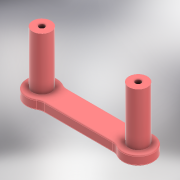
# Autodesk Inventor part: BRAÇO ROBÓTICO - Garra A2b - Pino
Saved by Autodesk Inventor 2021 (Build 250183000, 183)
## iProperties
Created: 2020-08-23
Part Number: BRAÇO ROBÓTICO - Garra A2b - Pino
Material: Plástico PC/ABS
Document SubType Name: Modeling
Designer: Araújo, I.
Mass: 0.348924 g
Surface Area: 10.9374 cm^2
Volume: 0.976633 cm^3
Density: 0.357273 g/cm^3
Appearance: Liso - Branco
Author: Araújo, I.
## iProperties of the stored document _3DPrint.ipt
Created: 2020-11-23
Part Number: _3DPrint
Material: Genérico
Document SubType Name: Modeling
Designer: Araújo, I.
Mass: 0.976633 g
Surface Area: 10.9374 cm^2
Volume: 0.976633 cm^3
Density: 1 g/cm^3
Appearance: Padrão
Author: Araújo, I.
Autodesk Inventor part; units mm, degrees
ref_plane "YZ Plane" through (0, 0, 0) normal (1, 0, 0) x (0, 1, 0)
ref_plane "XZ Plane" through (0, 0, 0) normal (0, 1, 0) x (-1, 0, 0)
ref_plane "XY Plane" through (0, 0, 0) normal (0, 0, 1) x (1, 0, 0)
sketch "Esboço1" plane through (0, 0, 0) normal (0, 1, 0) x (-1, 0, 0)
  arc A0 (-2.0603, -3.4286) -> (-2.0603, 3.4286) centre (0, 0) ccw
  arc A1 (-22.9397, 3.4286) -> (-22.9397, -3.4286) centre (-25, 0) ccw
  line L0 (-3.6056, -3) -> (-21.3944, -3)
  line L1 (-3.6056, 3) -> (-21.3944, 3)
  arc A2 (-2.0603, -3.4286) -> (-3.6056, -3) centre (-3.6056, -6) ccw
  arc A3 (-3.6056, 3) -> (-2.0603, 3.4286) centre (-3.6056, 6) ccw
  arc A4 (-21.3944, -3) -> (-22.9397, -3.4286) centre (-21.3944, -6) ccw
  arc A5 (-22.9397, 3.4286) -> (-21.3944, 3) centre (-21.3944, 6) ccw
  point P0 (-2.6458, -3)
  point P1 (-22.3542, -3)
  point P2 (-2.6458, 3)
  point P3 (-22.3542, 3)
  dimension "d3" = 6
  dimension "d5" = 3
  dimension "d11" = 25
  dimension "d13" = 4
  constraints: 16 point on circle, 8 tangent, 6 centre point, 4 end point, 4 equal radius, 4 point on line, 2 parallel, 1 coincident, 1 horizontal, 1 horizontal alignment
  measures "d3" distance between parallel lines of L1 L0
  measures "d5" radius of A2
  measures "d11" distance of A1.centre A0.centre
  measures "d13" radius of A0
extrude "Extrusão1" add sketch "Esboço1" along normal blind 2.5
fillet "Arredondamento1" radius 0.3 16 edges at (22.1962, 0, 3.1091) (29, 0, 0) (22.1962, 0, -3.1091) (12.5, 0, -3) (2.8038, 0, -3.1091) (-4, 0, 0) (2.8038, 0, 3.1091) (12.5, 0, 3) (22.1962, 2.5, 3.1091) (29, 2.5, 0) (22.1962, 2.5, -3.1091) (12.5, 2.5, -3) (2.8038, 2.5, -3.1091) (-4, 2.5, 0) (2.8038, 2.5, 3.1091) (12.5, 2.5, 3)
sketch "Esboço2" plane through (0, 2.5, 0) normal (0, 1, 0) x (1, 0, 0)
  circle A0 centre (0, 0) radius 2.4
  circle A1 centre (25, 0) radius 2.4
  arc A2 (23.0942, -3.1714) -> (23.0942, 3.1714) centre (25, 0) ccw projected
  dimension "d14" = 4.8
  constraints: 2 centre point, 2 coincident, 1 equal radius
  measures "d14" diameter of A0
extrude "Extrusão2" add sketch "Esboço2" along normal blind 13.7
sketch "Esboço3" plane through (0, 16.2, 0) normal (0, 1, 0) x (1, 0, 0)
  circle A0 centre (0, 0) radius 2.4 projected
  circle A1 centre (25, 0) radius 2.4 projected
  constraints: 2 coincident
hole "Furo1" at (0, 16.2, 0) at (25, 16.2, 0) direction (0, -1, 0) diameter 1.5 depth 10 tip angle 118
